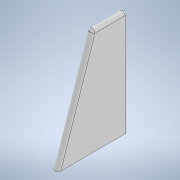
# Autodesk Inventor part: vertical_tail_surface
Saved by Autodesk Inventor 2021 (Build 250183000, 183)
## iProperties
Created: 2020-11-20
Part Number: vertical_tail_surface
Material: Generic
Document SubType Name: Modeling
Designer: Paco
Density: 1 g/cm^3
Appearance: Default
Author: Paco
Autodesk Inventor part; units mm, degrees
ref_plane "YZ Plane" through (0, 0, 0) normal (1, 0, 0) x (0, 1, 0)
ref_plane "XZ Plane" through (0, 0, 0) normal (0, 1, 0) x (-1, 0, 0)
ref_plane "XY Plane" through (0, 0, 0) normal (0, 0, 1) x (1, 0, 0)
sketch "Sketch1" plane through (0, 0, 0) normal (1, 0, 0) x (0, 1, 0)
  line L0 (-48.6957, 60.087) -> (-48.6957, -59.913)
  line L1 (-48.6957, -59.913) -> (131.3043, -59.913)
  line L2 (-48.6957, 60.087) -> (131.3043, 0.087)
  line L3 (131.3043, 0.087) -> (131.3043, -59.913)
  point P0 (0, 0)
  dimension "d0" = 120
  dimension "d1" = 60
  dimension "d2" = 180
  constraints: 8 end point, 1 parallel, 1 vertical
  measures "d0" distance of L0.start L0.end
  measures "d1" distance of L2.end L1.end
  measures "d2" distance of L0.end L1.end
extrude "Extrusion1" add sketch "Sketch1" along normal blind 10
fillet "Fillet1" radius 5 8 edges at (10, 41.3043, 30.087) (0, 41.3043, 30.087) (5, 131.3043, 0.087) (0, 131.3043, -29.913) (10, 131.3043, -29.913) (5, 131.3043, -59.913) (10, 41.3043, -59.913) (0, 41.3043, -59.913)
body "Solid1"
